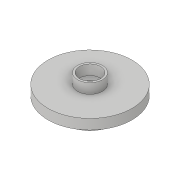
# Autodesk Inventor part: 30_CUBE_openSIM_Laser_FPC_mount
Saved by Autodesk Inventor 2019 (Build 230136000, 136)
## iProperties
Created: 2019-12-13
Part Number: 30_CUBE_openSIM_Laser_FPC_mount
Material: Generic
Document SubType Name: Modeling
Designer: diederichbenedict
Density: 1 g/cm^3
Appearance: Default
Author: diederichbenedict
Autodesk Inventor part; units mm, degrees
ref_plane "YZ Plane" through (0, 0, 0) normal (1, 0, 0) x (0, 1, 0)
ref_plane "XZ Plane" through (0, 0, 0) normal (0, 1, 0) x (-1, 0, 0)
ref_plane "XY Plane" through (0, 0, 0) normal (0, 0, 1) x (1, 0, 0)
sketch "Sketch1" plane through (0, 0, 0) normal (0, 1, 0) x (-1, 0, 0)
  circle A0 centre (0, 0) radius 12.5
  circle A1 centre (0, 0) radius 1.45
  dimension "d0" = 25
  dimension "d1" = 2.9
  constraints: 2 centre point, 2 coincident
  measures "d0" diameter of A0
  measures "d1" diameter of A1
extrude "Extrusion1" add sketch "Sketch1" along normal blind 3
sketch "Sketch2" plane through (0, 3, 0) normal (0, 1, 0) x (1, 0, 0)
  circle A0 centre (0, 0) radius 1.45 projected
  circle A1 centre (0, 0) radius 3.15
  circle A2 centre (0, 0) radius 3.7
  dimension "d4" = 6.3
  dimension "d5" = 7.4
  constraints: 2 centre point, 2 coincident
  measures "d4" diameter of A1
  measures "d5" diameter of A2
extrude "Extrusion2" add sketch "Sketch2" along normal blind 3 contours A2
sketch "Sketch3" plane through (0, 0, 0) normal (0, -1, 0) x (1, 0, 0)
  circle A0 centre (0, 0) radius 1.45 projected
  line L0 (-4.45, -4.45) -> (4.45, -4.45)
  line L1 (4.45, -4.45) -> (4.45, 4.45)
  line L2 (4.45, 4.45) -> (-4.45, 4.45)
  line L3 (-4.45, 4.45) -> (-4.45, -4.45)
  line L4 (-4.45, -4.45) -> (4.45, 4.45) construction
  line L5 (4.45, -4.45) -> (-4.45, 4.45) construction
  circle A1 centre (0, 0) radius 8.4362
  line L6 (-4.45, 1.45) -> (-8.3107, 1.45)
  line L7 (-4.45, -1.45) -> (-8.3107, -1.45)
  dimension "d8" = 8.9
  dimension "d9" = 8.9
  constraints: 16 end point, 3 parallel, 2 horizontal, 2 midpoint, 2 point on circle, 2 point on line, 1 centre point, 1 coincident, 1 perpendicular
  measures "d8" distance of L2.end L1.end
  measures "d9" distance of L1.end L0.end
extrude "Extrusion3" add sketch "Sketch3" along normal blind 3 contours L0 L1 L2 L3 L6 A1 L7
body "Solid1"
